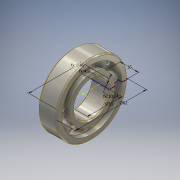
# Autodesk Inventor part: Подшипник-206
Saved by Autodesk Inventor 2016 (Build 200138000, 138)
## iProperties
Created: 2021-04-07
Part Number: Подшипник-206
Material: Типовые
Document SubType Name: Modeling
Designer: Лол
Density: 1 g/cm^3
Appearance: Титан — полированный
Author: Лол
Autodesk Inventor part; units mm, degrees
ref_plane "YZ Plane" through (0, 0, 0) normal (1, 0, 0) x (0, 1, 0)
ref_plane "XZ Plane" through (0, 0, 0) normal (0, 1, 0) x (-1, 0, 0)
ref_plane "XY Plane" through (0, 0, 0) normal (0, 0, 1) x (1, 0, 0)
sketch "Эскиз1" plane through (0, 0, 0) normal (0, 0, 1) x (1, 0, 0)
  line L0 (-11.9, 0) -> (11.9, 0) construction
  line L1 (0, -7.2) -> (0, 43.2) construction
  line L2 (-8, 31) -> (8, 31)
  line L3 (8, 15) -> (-8, 15)
  line L4 (-8, 31) -> (8, 31)
  line L5 (8, 31) -> (8, 26.2)
  line L6 (-8, 26.2) -> (-8, 31)
  line L7 (-8, 15) -> (8, 15)
  line L8 (8, 15) -> (8, 19.8)
  line L9 (-8, 19.8) -> (-8, 15)
  circle A0 centre (0, 23) radius 5.12
  line L10 (8, 26.2) -> (3.9968, 26.2)
  line L11 (-3.9968, 26.2) -> (-8, 26.2)
  line L12 (8, 19.8) -> (3.9968, 19.8)
  line L13 (-3.9968, 19.8) -> (-8, 19.8)
  line L14 (8, 31) -> (8, 26.2)
  line L15 (8, 19.8) -> (8, 15)
  line L16 (-8, 15) -> (-8, 19.8)
  line L17 (-8, 26.2) -> (-8, 31)
  line L18 (0, 28.12) -> (0, 17.88)
  point P0 (0, 0)
  dimension "D_" = 62
  dimension "d_" = 30
  dimension "D_w" = 10.24
  dimension "b" = 16
  dimension "S_" = 4.8
  dimension "d6" = 46
  constraints: 35 end point, 11 parallel, 6 point on circle, 4 perpendicular, 3 horizontal, 3 point on line, 2 equal length, 2 horizontal alignment, 1 centre point, 2 other
  measures "D_" diameter of L2 L0
  measures "d_" diameter of L3 L0
  measures "D_w" diameter of A0
  measures "b" distance of L2.start L2.end
  measures "S_" distance of L9.start L3.end
  measures "d6" diameter of A0.centre L0
revolve "Вращение1" add sketch "Эскиз1" angle 360 about axis through (-10, 0, 0) along (1, 0, 0) contours A0 L12 L8 L3 L9 L13
revolve "Вращение2" add sketch "Эскиз1" angle 360 about axis through (-10, 0, 0) along (1, 0, 0) separate body contours L2 L5 L10 A0 L11 L6
revolve "Вращение3" add sketch "Эскиз1" angle 360 about axis through (0, 28.12, 0) along (0, -1, 0) separate body picked at (2.0902, 24.0667) contours A0 L18
pattern_circular "Круговой массив1" count 8 over 360 about axis through (0, 0, 0) along (1, 0, 0) of "Вращение3" bodies 3
chamfer "Фаска4" distance 1 angle 45 4 edges at (8, -15, 0) (-8, -15, 0) (8, -31, 0) (-8, -31, 0)
equation "\"D_w\" = -0.32 * d_ + 0.32 * D_"
equation "\"S_\" = -0.15 * d_ + 0.15 * D_"
equation "\"d6\" = 0.5 * d_ + 0.5 * D_"
